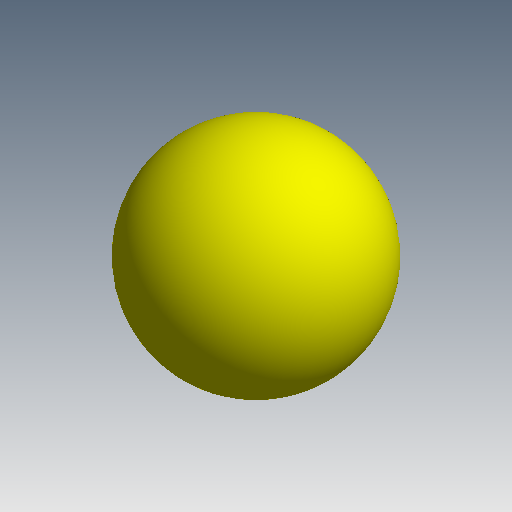
# Autodesk Inventor part: SKF_619/6-2Z_PART3
Saved by Autodesk Inventor 2020 (Build 240168000, 168)
## iProperties
Part Number: SKF_619/6-2Z_PART3
Material: Generic
Catalog Web Link: www.cadenas.de
Description: -Deep groove ball bearings
Vendor: SKF
Document SubType Name: Modeling
Designer: partserver
Manufacturer: SKF
Mass: 4 g
Surface Area: 0.178102 cm^2
Volume: 0.00706768 cm^3
Density: 1 g/cm^3
Appearance: PSOLRGB-192-192-192
Category: PARTsolutions
Company: SKF
PSOL_IDENT_0: {$CADENAS_DATA\23d-libs\skf\bearings_units_and_housings\ball_bearings\deep_groove_ball_bearings\bb1_
PSOL_IDENT_1: 001_101.prj},202 {VTYP=3D},{NB=SKF_619/6-2Z_PART3},{LINA=SKF_619/6-2Z_PART3},{NN=BB1_001_101_PART3},
PSOL_IDENT_2: {NOPRJ=TRUE},{DATE=20.09.2021 12:01:25},{GEOMDATE=07.09.2021 05:54:21},{VERSION=},{LINEID=9600},{WBV
PSOL_IDENT_3: AR=},{WBNUMERIC=}  {NB=SKF_619/6-2Z_PART3},{LINA=SKF_619/6-2Z_PART3},{KT=DUMMY},{DESIGNATION=619/6-2
PSOL_IDENT_4: Z},{R12=0.20},{DD=6.000},{D=15.000},{B=5.000},{C=},{CX=},{CXX=},{CA=0.000},{XXVARIANT=},{XXDESIGN=Si
PSOL_IDENT_5: ngle row},{XXSEALING=Shield on both sides},{DESIGN=dgbbw2z},{DESIGNIR=dgbbw2z},{VARIANT=},{DD1=8.20}
PSOL_IDENT_6: ,{DD2=},{DD2X=},{DD2A=0.00},{D1=11.70},{D1X=MIN},{D2=13},{D2A=13.00},{D3=},{D3X=},{D3A=0.000},{D4=},
PSOL_IDENT_7: {HH=MIN},{BB=MIN},{BBX=},{BBA=0.000},{FF=},{R0MAX=MIN},{R0=MIN},{PITCH=10.00},{DW=2.381},{DDAMIN=7.4
PSOL_IDENT_8: 00},{DDAMAX=8.000},{DDBMIN=MIN},{DDBMAX=MIN},{DBMIN=MIN},{DAMAX=13.600},{BBAMIN=MIN},{CAMAX=MIN},{RA
PSOL_IDENT_9: MAX=0.200},{LOAD1=0.884},{LOAD2=0.270},{LOAD3=0.011},{SPEED1=100000},{SPEED2=50000},{KR=0.020},{F0=6
PSOL_IDENT_10: .800},{Z=7},{II=1},{MASS=0.004},{BEARING=619/6-2Z},{RING=},{HELP=1.650},{HELP2=1.000},{DD1ALG=4.100}
PSOL_IDENT_11: ,{YALG=4.100},{PITCH1=10.000},{DW1=2.381},{YALG1=5.850},{HALG1=1.650},{SH=4.100},{CU=0.524},{HALG=1.
PSOL_IDENT_12: 1},{B1=0},{SHIELDHELP=2},{D4A=0.000},{FFA=0.000},{RS1=}
NB: SKF_619/6-2Z_PART3
NT: Deep groove ball bearings
NBSYN: SKF_$DESIGNATION._PART3
LINA: SKF_619/6-2Z_PART3
CATALOG: SKF
DESIGNATION: 619/6-2Z
R12: 0.2
DD: 6
D: 15
B: 5
D2: 13
LOAD1: 0.884
LOAD2: 0.27
LOAD3: 0.011
SPEED1: 100000
SPEED2: 50000
BEARING: 619/6-2Z
SUPPLIER: SKF
ARTICLENO: SKF_619/6-2Z_PART3
BOMINFO: SKF_619/6-2Z_PART3
CREATOR: CADENAS GmbH
Title: SKF_619/6-2Z_PART3
Author: Cadenas PARTsolutions
Comments: Deep groove ball bearings
Autodesk Inventor part; units mm, degrees
ref_plane "YZ Plane" through (0, 0, 0) normal (1, 0, 0) x (0, 1, 0)
ref_plane "XZ Plane" through (0, 0, 0) normal (0, 1, 0) x (-1, 0, 0)
ref_plane "XY Plane" through (0, 0, 0) normal (0, 0, 1) x (1, 0, 0)
sketch "Sketch_6" plane through (0, 0, 0) normal (0, 0, 1) x (1, 0, 0)
  line L0 (3.6905, 5) -> (1.3095, 5)
  arc A0 (3.6905, 5) -> (1.3095, 5) centre (2.5, 5) ccw
  line L1 (3.6905, 5) -> (1.3095, 5)
  dimension "d0" = 360
  constraints: 4 end point, 2 point on circle, 1 centre point
revolve "Revolution1" add sketch "Sketch_6" angle 360 about axis through (3.6905, 5, 0) along (1, 0, 0)
body "Solid1"
